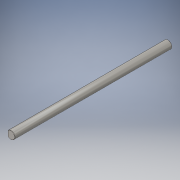
# Autodesk Inventor part: 634082
Saved by Autodesk Inventor 2016 SP1 (Build 200210100, 210)
## iProperties
Created: 2017-02-16
Part Number: 634082
Material: Stainless Steel
Document SubType Name: Modeling
Designer: 601898
Density: 8 g/cm^3
Appearance: Semi-Polished
Description: 1/4" Stainless Steel D-Shafting
Author: 601898
Title: 634082
Autodesk Inventor part; units mm, degrees
ref_plane "YZ Plane" through (0, 0, 0) normal (1, 0, 0) x (0, 1, 0)
ref_plane "XZ Plane" through (0, 0, 0) normal (0, 1, 0) x (-1, 0, 0)
ref_plane "XY Plane" through (0, 0, 0) normal (0, 0, 1) x (1, 0, 0)
sketch "Sketch1" plane through (0, 0, 0) normal (0, 0, 1) x (1, 0, 0)
  arc A0 (-2.4168, -2.0492) -> (-2.4168, 2.0492) centre (0, 0) ccw
  line L0 (-2.4168, 2.0492) -> (-2.4168, -2.0492)
  dimension "d0" = 6.3373
  dimension "d1" = 5.5855
  constraints: 2 end point, 2 point on circle, 1 centre point, 1 coincident, 1 vertical
  measures "d0" diameter of A0
extrude "Extrusion1" add sketch "Sketch1" along normal blind 127
chamfer "Chamfer1" distance 0.254 angle 45 6 edges at (-2.4168, 2.0492, 63.5) (-2.4168, -2.0492, 63.5) (-2.4168, 0, 127) (3.1687, 0, 0) (-2.4168, 0, 0) (3.1687, 0, 127)
body "Solid1"
